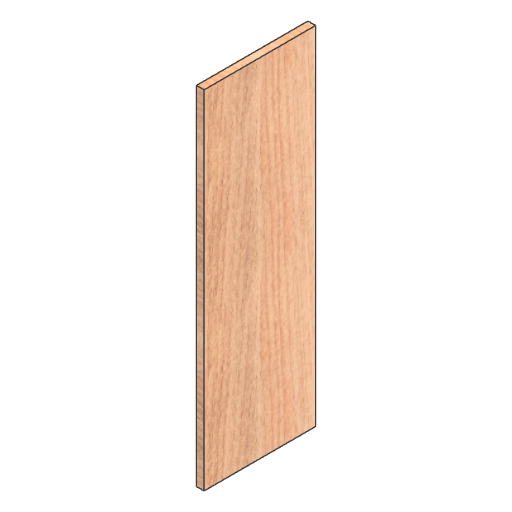
# Autodesk Inventor part: CUT PART H-01
Saved by Autodesk Inventor 2023.2 (Build 272271000, 271)
## iProperties
Created: 2022-11-02
Part Number: CUT PART H-01
Material: Wood (Birch)
Document SubType Name: Modeling
Designer: GUT
Density: 0.55 g/cm^3
Appearance: Birch - Natural Polished
Mass: 629.475 g
Surface Area: 2080.3 cm^2
Volume: 1144.5 cm^3
d1: 175,000 mm
Author: GUT
Autodesk Inventor part; units mm, degrees
ref_plane "YZ Plane" through (0, 0, 0) normal (1, 0, 0) x (0, 1, 0)
ref_plane "XZ Plane" through (0, 0, 0) normal (0, 1, 0) x (-1, 0, 0)
ref_plane "XY Plane" through (0, 0, 0) normal (0, 0, 1) x (1, 0, 0)
sketch "Sketch1" plane through (0, 0, 0) normal (1, 0, 0) x (0, 1, 0)
  line L0 (133.5393, 19.0641) -> (678.5393, 19.0641)
  line L1 (678.5393, 19.0641) -> (678.5393, -155.9359)
  line L2 (678.5393, -155.9359) -> (133.5393, -155.9359)
  line L3 (133.5393, -155.9359) -> (133.5393, 19.0641)
  point P0 (0, 0)
  dimension "b" = 545
  dimension "d1" = 175
  constraints: 8 end point, 2 parallel, 1 horizontal, 1 perpendicular
  measures "b" distance of L1.end L2.end
  measures "d1" distance of L0.end L1.end
extrude "Extrusion1" add sketch "Sketch1" along normal blind 12
body "Solid1"
